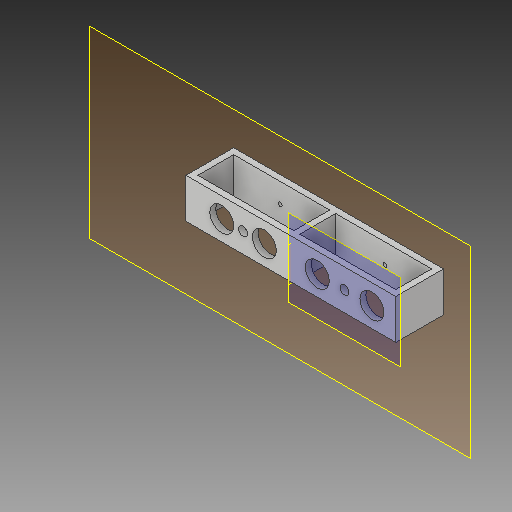
# Autodesk Inventor part: buttonHolder
Saved by Autodesk Inventor 2017.3 (Build 213257000, 257)
## iProperties
Created: 2021-12-06
Part Number: buttonHolder
Material: Generic
Document SubType Name: Modeling
Designer: TEOS
Density: 1 g/cm^3
Appearance: Default
Author: TEOS
Autodesk Inventor part; units mm, degrees
ref_plane "YZ Plane" through (0, 0, 0) normal (1, 0, 0) x (0, 1, 0)
ref_plane "XZ Plane" through (0, 0, 0) normal (0, 1, 0) x (-1, 0, 0)
ref_plane "XY Plane" through (0, 0, 0) normal (0, 0, 1) x (1, 0, 0)
ref_plane "Work Plane2" through (56.5, 19.5, 24) normal (0, 0, -1) x (-1, 0, 0)
sketch "Sketch2" plane through (56.5, 19.5, 24) normal (0, 0, -1) x (-1, 0, 0)
  circle A0 centre (-13.7, 0) radius 2.5
  circle A1 centre (13.7, 0) radius 2.5
  line L0 (25.7, -17.7) -> (25.7, 17.7)
  line L1 (25.7, 17.7) -> (-25.7, 17.7)
  line L2 (-25.7, 17.7) -> (-25.7, -17.7)
  line L3 (-25.7, -17.7) -> (25.7, -17.7)
  arc A2 (79.7, 4.408) -> (68.0785, -17.7) centre (105, -23) ccw
  line L4 (79.7, 4.408) -> (79.7, 17.7)
  line L5 (79.7, 17.7) -> (28.3, 17.7)
  line L6 (28.3, 17.7) -> (28.3, -17.7)
  line L7 (28.3, -17.7) -> (68.0785, -17.7)
  line L8 (-25.7, -10) -> (79.7, -10)
  line L9 (79.7, -10) -> (79.7, 10)
  line L10 (79.7, 10) -> (-25.7, 10)
  line L11 (-25.7, 10) -> (-25.7, -10)
  circle A3 centre (-13.7, 0) radius 6
  circle A4 centre (13.7, 0) radius 6
  circle A5 centre (40.3, 0) radius 6
  circle A6 centre (61.7, 0) radius 6
  line L12 (-13.7, 0) -> (13.7, 0)
  line L13 (40.3, 0) -> (61.7, 0)
  circle A7 centre (0, 0) radius 2.25
  circle A8 centre (51, 0) radius 2.25
  line L14 (4.5099, -3.2615) -> (2.8081, -0.5216)
  line L15 (2.8081, -0.5216) -> (1.1404, -3.2615)
  line L16 (1.1404, -3.2615) -> (0.074, -3.2615)
  line L17 (0.074, -3.2615) -> (2.2352, 0.2328)
  line L18 (2.2352, 0.2328) -> (0.0059, 3.7385)
  line L19 (0.0059, 3.7385) -> (1.0099, 3.7385)
  line L20 (1.0099, 3.7385) -> (2.7458, 0.9476)
  line L21 (2.7458, 0.9476) -> (4.4475, 3.7385)
  line L22 (4.4475, 3.7385) -> (5.514, 3.7385)
  line L23 (5.514, 3.7385) -> (3.3244, 0.1875)
  line L24 (3.3244, 0.1875) -> (5.514, -3.2615)
  line L25 (5.514, -3.2615) -> (4.5099, -3.2615)
  line L26 (-2.3823, -2.4333) -> (-0.0338, -2.4333)
  line L27 (-0.0338, -2.4333) -> (-0.0338, -3.2615)
  line L28 (-0.0338, -3.2615) -> (-5.6611, -3.2615)
  line L29 (-5.6611, -3.2615) -> (-5.6611, -2.4333)
  line L30 (-5.6611, -2.4333) -> (-3.3126, -2.4333)
  line L31 (-3.3126, -2.4333) -> (-3.3126, 3.7385)
  line L32 (-3.3126, 3.7385) -> (-2.3823, 3.7385)
  line L33 (-2.3823, 3.7385) -> (-2.3823, -2.4333)
  arc A9 (42.6087, -0.959) -> (42.3892, -1.3731) centre (40.3, 0) ccw
  arc A10 (59.4794, -1.1484) -> (60.4698, 2.1764) centre (61.7, 0) ccw
  line L34 (57.8929, -1.3844) -> (57.5298, -1.3844)
  spline S0 degree 3 poles (57.5298, -1.3844) (57.5237, -1.3081) (57.5086, -1.2288) (57.4558, -1.1142) (57.4282, -1.0735) (57.3717, -1.0212) (57.3384, -0.995) (57.2167, -0.9422) (57.1455, -0.9254) (56.9893, -0.9013) (56.8956, -0.8966) (56.8066, -0.8966) knots 0 0 0 0 0.345306 0.345306 0.567996 0.567996 0.69168 0.69168 0.826183 0.826183 1 1 1 1
  line L35 (56.8066, -0.8966) -> (56.8066, -0.5761)
  line L36 (56.8066, -0.5761) -> (57.4419, -0.5761)
  line L37 (57.4419, -0.5761) -> (57.4419, 1.7695)
  line L38 (57.4419, 1.7695) -> (56.8066, 1.7695)
  line L39 (56.8066, 1.7695) -> (56.8066, 2.1269)
  line L40 (56.8066, 2.1269) -> (58.514, 2.1269)
  line L41 (58.514, 2.1269) -> (58.514, 1.7695)
  line L42 (58.514, 1.7695) -> (57.8929, 1.7695)
  line L43 (57.8929, 1.7695) -> (57.8929, -1.3844)
  spline S1 degree 3 poles (45.7308, 1.7809) (45.6428, 1.7809) (45.5609, 1.7718) (45.4737, 1.739) (45.4331, 1.721) (45.3624, 1.6543) (45.3386, 1.6213) (45.3196, 1.5852) knots 0 0 0 0 0.620283 0.620283 0.840472 0.840472 1 1 1 1
  spline S2 degree 3 poles (45.3196, 1.5852) (45.285, 1.5198) (45.2647, 1.448) (45.2437, 1.3061) (45.2345, 1.1849) (45.2345, 0.9981) knots 0 0 0 0 0.515302 0.515302 1 1 1 1
  line L44 (45.2345, 0.9981) -> (45.2345, -0.4995)
  line L45 (45.2345, -0.4995) -> (44.792, -0.4995)
  line L46 (44.792, -0.4995) -> (44.792, 1.2051)
  spline S3 degree 3 poles (44.792, 1.2051) (44.792, 1.3545) (44.8067, 1.5155) (44.8672, 1.6957) (44.8911, 1.7601) (44.958, 1.877) (44.9913, 1.9233) (45.0302, 1.9652) knots 0 0 0 0 0.681131 0.681131 0.864505 0.864505 1 1 1 1
  spline S4 degree 3 poles (45.0302, 1.9652) (45.0905, 2.0317) (45.1609, 2.0847) (45.3085, 2.1538) (45.3745, 2.1714) (45.4853, 2.1945) (45.5496, 2.2006) (45.6145, 2.2006) knots 0 0 0 0 0.34299 0.34299 0.623064 0.623064 1 1 1 1
  spline S5 degree 3 poles (45.6145, 2.2006) (45.7367, 2.2006) (45.856, 2.1806) (46.1082, 2.0762) (46.2634, 1.9672) (46.4115, 1.8376) knots 0 0 0 0 0.447538 0.447538 1 1 1 1
  line L47 (46.4115, 1.8376) -> (46.4115, 2.1269)
  line L48 (46.4115, 2.1269) -> (46.854, 2.1269)
  line L49 (46.854, 2.1269) -> (46.854, -0.4995)
  line L50 (46.854, -0.4995) -> (46.4115, -0.4995)
  line L51 (46.4115, -0.4995) -> (46.4115, 1.4632)
  spline S6 degree 3 poles (46.4115, 1.4632) (46.309, 1.5525) (46.1968, 1.6275) (46.0461, 1.7035) (45.9801, 1.7358) (45.8432, 1.7724) (45.7873, 1.7809) (45.7308, 1.7809) knots 0 0 0 0 0.713371 0.713371 0.885673 0.885673 1 1 1 1
  spline S7 degree 3 poles (51.8516, 1.6844) (51.7705, 1.7209) (51.6843, 1.748) (51.5493, 1.7794) (51.4479, 1.8007) (51.3127, 1.8007) knots 0 0 0 0 0.641471 0.641471 1 1 1 1
  spline S8 degree 3 poles (51.3127, 1.8007) (51.1845, 1.8007) (51.0556, 1.7828) (50.8451, 1.6988) (50.7638, 1.6466) (50.6381, 1.5232) (50.5772, 1.4464) (50.4997, 1.2649) (50.4792, 1.1913) (50.4509, 1.032) (50.4448, 0.945) (50.4448, 0.8591) knots 0 0 0 0 0.314267 0.314267 0.555468 0.555468 0.746025 0.746025 0.865107 0.865107 1 1 1 1
  line L52 (50.4448, 0.8591) -> (52.2628, 0.8591)
  line L53 (52.2628, 0.8591) -> (52.2628, 0.618)
  spline S9 degree 3 poles (52.2628, 0.618) (52.2628, 0.4424) (52.2453, 0.2525) (52.1718, 0.0405) (52.143, -0.0344) (52.0602, -0.1744) (52.0187, -0.2302) (51.9707, -0.2811) knots 0 0 0 0 0.67479 0.67479 0.860065 0.860065 1 1 1 1
  spline S10 degree 3 poles (51.9707, -0.2811) (51.893, -0.3652) (51.8025, -0.4318) (51.617, -0.5165) (51.5377, -0.5373) (51.3865, -0.5664) (51.2983, -0.5733) (51.2106, -0.5733) knots 0 0 0 0 0.354979 0.354979 0.632418 0.632418 1 1 1 1
  spline S11 degree 3 poles (51.2106, -0.5733) (51.0481, -0.5733) (50.8885, -0.5476) (50.6078, -0.4322) (50.4929, -0.3547) (50.3003, -0.1657) (50.202, -0.0414) (50.0813, 0.2355) (50.0497, 0.3439) (50.0062, 0.5775) (49.9966, 0.7031) (49.9966, 0.8279) knots 0 0 0 0 0.273507 0.273507 0.511012 0.511012 0.727836 0.727836 0.857042 0.857042 1 1 1 1
  spline S12 degree 3 poles (49.9966, 0.8279) (49.9966, 1.0393) (50.0239, 1.2553) (50.1545, 1.5922) (50.2316, 1.7178) (50.4061, 1.8994) (50.5129, 1.991) (50.7696, 2.1065) (50.8695, 2.1363) (51.0857, 2.1775) (51.2024, 2.1865) (51.3183, 2.1865) knots 0 0 0 0 0.358444 0.358444 0.612146 0.612146 0.785167 0.785167 0.886845 0.886845 1 1 1 1
  spline S13 degree 3 poles (51.3183, 2.1865) (51.4021, 2.1865) (51.4991, 2.1826) (51.6606, 2.1542) (51.7381, 2.1348) (51.8147, 2.1127) knots 0 0 0 0 0.514065 0.514065 1 1 1 1
  spline S14 degree 3 poles (51.8147, 2.1127) (51.8833, 2.0934) (51.9554, 2.0677) (52.0547, 2.0289) (52.1398, 1.9957) (52.2146, 1.9652) knots 0 0 0 0 0.667879 0.667879 1 1 1 1
  line L54 (52.2146, 1.9652) -> (52.2146, 1.4831)
  line L55 (52.2146, 1.4831) -> (52.1891, 1.4831)
  spline S15 degree 3 poles (52.1891, 1.4831) (52.1478, 1.5178) (52.099, 1.5503) (52.0076, 1.6054) (51.9453, 1.6398) (51.8516, 1.6844) knots 0 0 0 0 0.503966 0.503966 1 1 1 1
  line L56 (55.102, 0.479) -> (54.4666, -0.4995)
  line L57 (54.4666, -0.4995) -> (53.9249, -0.4995)
  line L58 (53.9249, -0.4995) -> (54.8268, 0.825)
  line L59 (54.8268, 0.825) -> (53.9164, 2.1269)
  line L60 (53.9164, 2.1269) -> (54.4184, 2.1269)
  line L61 (54.4184, 2.1269) -> (55.0736, 1.1399)
  line L62 (55.0736, 1.1399) -> (55.7118, 2.1269)
  line L63 (55.7118, 2.1269) -> (56.2535, 2.1269)
  line L64 (56.2535, 2.1269) -> (55.3487, 0.7967)
  line L65 (55.3487, 0.7967) -> (56.2535, -0.4995)
  line L66 (56.2535, -0.4995) -> (55.7515, -0.4995)
  line L67 (55.7515, -0.4995) -> (55.102, 0.479)
  line L68 (47.9375, -0.4995) -> (47.495, -0.4995)
  line L69 (47.495, -0.4995) -> (47.495, 2.1269)
  line L70 (47.495, 2.1269) -> (47.9375, 2.1269)
  line L71 (47.9375, 2.1269) -> (47.9375, 0.1642)
  spline S16 degree 3 poles (47.9375, 0.1642) (48.0425, 0.0752) (48.1563, -0.0036) (48.3085, -0.0803) (48.3714, -0.1108) (48.5059, -0.1457) (48.5616, -0.1535) (48.6182, -0.1535) knots 0 0 0 0 0.713918 0.713918 0.883625 0.883625 1 1 1 1
  spline S17 degree 3 poles (48.6182, -0.1535) (48.7, -0.1535) (48.7817, -0.1446) (48.8974, -0.0998) (48.93, -0.076) (48.9847, -0.0271) (49.0096, 0.0057) (49.0294, 0.0422) knots 0 0 0 0 0.380701 0.380701 0.649134 0.649134 1 1 1 1
  spline S18 degree 3 poles (49.0294, 0.0422) (49.0561, 0.0912) (49.073, 0.1478) (49.1133, 0.3489) (49.1145, 0.5537) (49.1145, 0.6293) knots 0 0 0 0 0.271467 0.271467 1 1 1 1
  line L72 (49.1145, 0.6293) -> (49.1145, 2.1269)
  line L73 (49.1145, 2.1269) -> (49.557, 2.1269)
  line L74 (49.557, 2.1269) -> (49.557, 0.4223)
  spline S19 degree 3 poles (49.557, 0.4223) (49.557, 0.2581) (49.5382, 0.0862) (49.4352, -0.1948) (49.3743, -0.2801) (49.2563, -0.408) (49.1824, -0.4621) (49.0432, -0.5259) (48.9864, -0.5435) (48.8642, -0.5679) (48.7993, -0.5733) (48.7345, -0.5733) knots 0 0 0 0 0.2477 0.2477 0.450945 0.450945 0.686188 0.686188 0.836628 0.836628 1 1 1 1
  spline S20 degree 3 poles (48.7345, -0.5733) (48.6109, -0.5733) (48.4919, -0.5502) (48.2777, -0.4606) (48.1258, -0.3769) (47.9375, -0.2074) knots 0 0 0 0 0.532257 0.532257 1 1 1 1
  line L75 (47.9375, -0.2074) -> (47.9375, -0.4995)
  line L76 (42.6087, -0.959) -> (42.852, -0.959)
  line L77 (42.852, -0.959) -> (42.852, 2.1269)
  line L78 (42.852, 2.1269) -> (43.3171, 2.1269)
  line L79 (43.3171, 2.1269) -> (43.3171, -0.959)
  line L80 (43.3171, -0.959) -> (44.4913, -0.959)
  line L81 (44.4913, -0.959) -> (44.4913, -1.3731)
  line L82 (44.4913, -1.3731) -> (42.3892, -1.3731)
  spline S21 degree 3 poles (59.4794, -1.1484) (59.3969, -1.0576) (59.3421, -0.9609) (59.2272, -0.7174) (59.1797, -0.5284) (59.1114, -0.1119) (59.0983, 0.1408) (59.0983, 0.3797) knots 0 0 0 0 0.169073 0.169073 0.529013 0.529013 1 1 1 1
  spline S22 degree 3 poles (59.0983, 0.3797) (59.0983, 0.7645) (59.1335, 1.1554) (59.3174, 1.6919) (59.4043, 1.8129) (59.536, 1.9692) (59.6237, 2.0404) (59.7982, 2.1301) (59.8747, 2.1564) (60.0407, 2.1927) (60.1298, 2.2006) (60.2187, 2.2006) knots 0 0 0 0 0.258939 0.258939 0.435748 0.435748 0.663533 0.663533 0.824156 0.824156 1 1 1 1
  spline S23 degree 3 poles (60.2187, 2.2006) (60.3032, 2.2006) (60.3875, 2.1934) (60.4698, 2.1764) knots 0 0 0 0 1 1 1 1
  point P0 (56.5, -19.5)
  dimension "d0" = 20
  dimension "d1" = 10
  dimension "d2" = 12
  dimension "d3" = 12
  dimension "d4" = 12
  dimension "d5" = 12
  dimension "d6" = 4.5
  dimension "d7" = 4.5
  constraints: 12 end point, 6 centre point, 3 horizontal, 2 coincident, 2 midpoint, 2 parallel, 2 point on line, 1 perpendicular
  measures "d0" distance between parallel lines of L10 L8
  measures "d1" distance from line of L8 A0.centre
  measures "d2" diameter of A3
  measures "d3" diameter of A4
  measures "d4" diameter of A5
  measures "d5" diameter of A6
  measures "d6" diameter of A7
  measures "d7" diameter of A8
extrude "Extrusion1" add sketch "Sketch2" along normal blind 3 contours L8 L2 L10 L0 | L0 L10 L6 L8 | L6 L10 L4 A2 L8 | A2 L9 L8 | A5 S6 L51 L13 | A5 S5 L47 L48 L49 L13 L51 S6 | L13 L49 L50 L51 | A6 L64 L65 L13 L67 L56 L58 L59 L60 L61 L62 L63 | L67 L13 A6 | A6 L65 L64 | L13 L56 L67 | L56 L57 L58 L13 | L31 L32 L33 L12 | L12 L33 L26 L27 L28 L29 L30 L31 | L18 L19 L20 L21 L22 L23 L24 L12 A7 | A7 L12 L24 L25 L14 L15 L16 L17 | L69 L70 L71 S16 L13 | L13 S16 S17 A8 S19 S20 L75 L68 L69 | L13 A8 S17 S16 | L72 L73 L74 A8 | S13 S14 L54 A8
sketch "Sketch3" plane through (-23.2, 9.5, 24) normal (-1, 0, 0) x (0, 0, 1)
  line L0 (-3, 0) -> (-3, 20) projected
  line L1 (-24, 27.5) -> (-24, -46.5) projected
  line L2 (-3, 20) -> (-24, 20)
  line L3 (-3, 0) -> (-24, 0)
  point P0 (-24, -9.5)
  constraints: 4 end point, 2 point on line, 1 horizontal, 1 perpendicular
extrude "Extrusion2" add sketch "Sketch3" against normal blind 3
sketch "Sketch4" plane through (82.2, 9.5, 24) normal (1, 0, 0) x (0, 0, -1)
  line L0 (3, 0) -> (3, 20) projected
  line L1 (3, 0) -> (24, 0) projected
  line L2 (24, 0) -> (24, 20) projected
  line L3 (24, 20) -> (3, 20) projected
  point P0 (24, -9.5)
extrude "Extrusion3" add sketch "Sketch4" against normal blind 3
ref_plane "Work Plane3" through (29.5, 9.5, 24) normal (1, 0, 0) x (0, 0, -1)
sketch "Sketch5" plane through (29.5, 9.5, 24) normal (1, 0, 0) x (0, 0, -1)
  line L0 (3, 0) -> (3, 20) projected
  line L1 (3, 0) -> (24, 0) projected
  line L2 (24, 0) -> (24, 20) projected
  line L3 (24, 20) -> (3, 20) projected
  point P0 (24, -9.5)
extrude "Extrusion4" add sketch "Sketch5" along normal mid plane 3
ref_plane "Work Plane4" through (0, 0, 0) normal (0, 0, 1) x (1, 0, 0)
sketch "Sketch6" plane through (0, 0, 0) normal (0, 0, 1) x (1, 0, 0)
  line L0 (79.2, 29.5) -> (79.2, 9.5) projected
  line L1 (79.2, 29.5) -> (-20.2, 29.5)
  line L2 (-20.2, 29.5) -> (-20.2, 9.5)
  line L3 (-20.2, 9.5) -> (79.2, 9.5)
  line L4 (79.2, 9.5) -> (79.2, 29.5)
  point P0 (0, 0)
  constraints: 8 end point, 2 parallel, 2 point on line, 1 horizontal, 1 perpendicular
extrude "Extrusion5" add sketch "Sketch6" along normal blind 3
sketch "Sketch7" plane through (82.2, 9.5, 0) normal (0, 0, -1) x (-1, 0, 0)
  circle A0 centre (87.4, 10) radius 6 projected
  circle A1 centre (66, 10) radius 6 projected
  circle A2 centre (76.7, 10) radius 2.25 projected
  circle A3 centre (39.4, 10) radius 6 projected
  circle A4 centre (12, 10) radius 6 projected
  circle A5 centre (25.7, 10) radius 2.25 projected
  line L0 (0, 0) -> (105.4, 0) projected
  line L1 (0, 20) -> (0, 0) projected
  line L2 (105.4, 20) -> (0, 20) projected
  line L3 (105.4, 0) -> (105.4, 20) projected
  line L4 (0, 0) -> (0, 20) projected
  line L5 (0, 20) -> (52.7, 0) construction
  line L6 (0, 0) -> (105.4, 0) projected
  line L7 (52.7, 0) -> (105.4, 20) construction
  line L8 (105.4, 20) -> (105.4, 0) projected
  line L9 (52.7, 20) -> (105.4, 0) construction
  line L10 (0, 0) -> (52.7, 20) construction
  point P0 (82.2, -9.5)
  point P1 (26.35, 10)
  point P2 (79.05, 10)
  constraints: 8 end point, 4 midpoint, 1 parallel
hole "Hole1" at (55.85, 19.5, 0) at (3.15, 19.5, 0) direction (0, 0, 1) diameter 2 depth 8 tip angle 118
body "Solid1"
